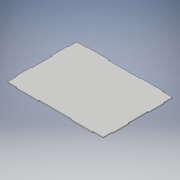
# Autodesk Inventor part: case_roof
Saved by Autodesk Inventor 2019 (Build 230136000, 136)
## iProperties
Created: 2019-07-12
Part Number: case_roof
Material: Generic
Document SubType Name: Modeling
Designer: Lino P
Density: 1 g/cm^3
Appearance: Default
Author: Lino P
Autodesk Inventor part; units mm, degrees
ref_plane "YZ Plane" through (0, 0, 0) normal (1, 0, 0) x (0, 1, 0)
ref_plane "XZ Plane" through (0, 0, 0) normal (0, 1, 0) x (-1, 0, 0)
ref_plane "XY Plane" through (0, 0, 0) normal (0, 0, 1) x (1, 0, 0)
sketch "Sketch1" plane through (0, 0, 0) normal (0, 0, 1) x (1, 0, 0)
  line L0 (0, 0) -> (27, 0)
  line L1 (27, 0) -> (27, 30.2)
  line L2 (27, 30.2) -> (0, 30.2)
  line L3 (0, 30.2) -> (0, 0)
  circle A0 centre (13.5, 15.1) radius 10.85
  circle A1 centre (4.1, 4.2) radius 1.3
  circle A2 centre (22.9, 26) radius 1.3
  line L4 (21.6, 26) -> (24.2, 26) construction
  line L5 (22.9, 26) -> (22.9, 27.3) construction
  line L6 (4.1, 4.2) -> (2.8, 4.2) construction
  line L7 (4.1, 4.2) -> (4.1, 2.9) construction
  line L8 (45, 0) -> (72, 0)
  line L9 (72, 0) -> (72, 30.2)
  line L10 (72, 30.2) -> (45, 30.2)
  line L11 (45, 30.2) -> (45, 0)
  circle A3 centre (58.5, 15.1) radius 10.85
  circle A4 centre (49.1, 4.2) radius 1.3
  circle A5 centre (67.9, 26) radius 1.3
  line L12 (66.6, 26) -> (69.2, 26) construction
  line L13 (67.9, 26) -> (67.9, 27.3) construction
  line L14 (49.1, 4.2) -> (47.8, 4.2) construction
  line L15 (49.1, 4.2) -> (49.1, 2.9) construction
  line L16 (90, 0) -> (117, 0)
  line L17 (117, 0) -> (117, 30.2)
  line L18 (117, 30.2) -> (90, 30.2)
  line L19 (90, 30.2) -> (90, 0)
  circle A6 centre (103.5, 15.1) radius 10.85
  circle A7 centre (94.1, 4.2) radius 1.3
  circle A8 centre (112.9, 26) radius 1.3
  line L20 (111.6, 26) -> (114.2, 26) construction
  line L21 (112.9, 26) -> (112.9, 27.3) construction
  line L22 (94.1, 4.2) -> (92.8, 4.2) construction
  line L23 (94.1, 4.2) -> (94.1, 2.9) construction
  line L24 (135, 0) -> (162, 0)
  line L25 (162, 0) -> (162, 30.2)
  line L26 (162, 30.2) -> (135, 30.2)
  line L27 (135, 30.2) -> (135, 0)
  circle A9 centre (148.5, 15.1) radius 10.85
  circle A10 centre (139.1, 4.2) radius 1.3
  circle A11 centre (157.9, 26) radius 1.3
  line L28 (156.6, 26) -> (159.2, 26) construction
  line L29 (157.9, 26) -> (157.9, 27.3) construction
  line L30 (139.1, 4.2) -> (137.8, 4.2) construction
  line L31 (139.1, 4.2) -> (139.1, 2.9) construction
  line L32 (180, 0) -> (207, 0)
  line L33 (207, 0) -> (207, 30.2)
  line L34 (207, 30.2) -> (180, 30.2)
  line L35 (180, 30.2) -> (180, 0)
  circle A12 centre (193.5, 15.1) radius 10.85
  circle A13 centre (184.1, 4.2) radius 1.3
  circle A14 centre (202.9, 26) radius 1.3
  line L36 (201.6, 26) -> (204.2, 26) construction
  line L37 (202.9, 26) -> (202.9, 27.3) construction
  line L38 (184.1, 4.2) -> (182.8, 4.2) construction
  line L39 (184.1, 4.2) -> (184.1, 2.9) construction
  line L40 (225, 0) -> (252, 0)
  line L41 (252, 0) -> (252, 30.2)
  line L42 (252, 30.2) -> (225, 30.2)
  line L43 (225, 30.2) -> (225, 0)
  circle A15 centre (238.5, 15.1) radius 10.85
  circle A16 centre (229.1, 4.2) radius 1.3
  circle A17 centre (247.9, 26) radius 1.3
  line L44 (246.6, 26) -> (249.2, 26) construction
  line L45 (247.9, 26) -> (247.9, 27.3) construction
  line L46 (229.1, 4.2) -> (227.8, 4.2) construction
  line L47 (229.1, 4.2) -> (229.1, 2.9) construction
  line L48 (270, 0) -> (297, 0)
  line L49 (297, 0) -> (297, 30.2)
  line L50 (297, 30.2) -> (270, 30.2)
  line L51 (270, 30.2) -> (270, 0)
  circle A18 centre (283.5, 15.1) radius 10.85
  circle A19 centre (274.1, 4.2) radius 1.3
  circle A20 centre (292.9, 26) radius 1.3
  line L52 (291.6, 26) -> (294.2, 26) construction
  line L53 (292.9, 26) -> (292.9, 27.3) construction
  line L54 (274.1, 4.2) -> (272.8, 4.2) construction
  line L55 (274.1, 4.2) -> (274.1, 2.9) construction
  line L56 (315, 0) -> (342, 0)
  line L57 (342, 0) -> (342, 30.2)
  line L58 (342, 30.2) -> (315, 30.2)
  line L59 (315, 30.2) -> (315, 0)
  circle A21 centre (328.5, 15.1) radius 10.85
  circle A22 centre (319.1, 4.2) radius 1.3
  circle A23 centre (337.9, 26) radius 1.3
  line L60 (336.6, 26) -> (339.2, 26) construction
  line L61 (337.9, 26) -> (337.9, 27.3) construction
  line L62 (319.1, 4.2) -> (317.8, 4.2) construction
  line L63 (319.1, 4.2) -> (319.1, 2.9) construction
  line L64 (0, -60) -> (27, -60)
  line L65 (27, -60) -> (27, -29.8)
  line L66 (27, -29.8) -> (0, -29.8)
  line L67 (0, -29.8) -> (0, -60)
  circle A24 centre (13.5, -44.9) radius 10.85
  circle A25 centre (4.1, -55.8) radius 1.3
  circle A26 centre (22.9, -34) radius 1.3
  line L68 (21.6, -34) -> (24.2, -34) construction
  line L69 (22.9, -34) -> (22.9, -32.7) construction
  line L70 (4.1, -55.8) -> (2.8, -55.8) construction
  line L71 (4.1, -55.8) -> (4.1, -57.1) construction
  line L72 (45, -60) -> (72, -60)
  line L73 (72, -60) -> (72, -29.8)
  line L74 (72, -29.8) -> (45, -29.8)
  line L75 (45, -29.8) -> (45, -60)
  circle A27 centre (58.5, -44.9) radius 10.85
  circle A28 centre (49.1, -55.8) radius 1.3
  circle A29 centre (67.9, -34) radius 1.3
  line L76 (66.6, -34) -> (69.2, -34) construction
  line L77 (67.9, -34) -> (67.9, -32.7) construction
  line L78 (49.1, -55.8) -> (47.8, -55.8) construction
  line L79 (49.1, -55.8) -> (49.1, -57.1) construction
  line L80 (90, -60) -> (117, -60)
  line L81 (117, -60) -> (117, -29.8)
  line L82 (117, -29.8) -> (90, -29.8)
  line L83 (90, -29.8) -> (90, -60)
  circle A30 centre (103.5, -44.9) radius 10.85
  circle A31 centre (94.1, -55.8) radius 1.3
  circle A32 centre (112.9, -34) radius 1.3
  line L84 (111.6, -34) -> (114.2, -34) construction
  line L85 (112.9, -34) -> (112.9, -32.7) construction
  line L86 (94.1, -55.8) -> (92.8, -55.8) construction
  line L87 (94.1, -55.8) -> (94.1, -57.1) construction
  line L88 (135, -60) -> (162, -60)
  line L89 (162, -60) -> (162, -29.8)
  line L90 (162, -29.8) -> (135, -29.8)
  line L91 (135, -29.8) -> (135, -60)
  circle A33 centre (148.5, -44.9) radius 10.85
  circle A34 centre (139.1, -55.8) radius 1.3
  circle A35 centre (157.9, -34) radius 1.3
  line L92 (156.6, -34) -> (159.2, -34) construction
  line L93 (157.9, -34) -> (157.9, -32.7) construction
  line L94 (139.1, -55.8) -> (137.8, -55.8) construction
  line L95 (139.1, -55.8) -> (139.1, -57.1) construction
  line L96 (180, -60) -> (207, -60)
  line L97 (207, -60) -> (207, -29.8)
  line L98 (207, -29.8) -> (180, -29.8)
  line L99 (180, -29.8) -> (180, -60)
  circle A36 centre (193.5, -44.9) radius 10.85
  circle A37 centre (184.1, -55.8) radius 1.3
  circle A38 centre (202.9, -34) radius 1.3
  line L100 (201.6, -34) -> (204.2, -34) construction
  line L101 (202.9, -34) -> (202.9, -32.7) construction
  line L102 (184.1, -55.8) -> (182.8, -55.8) construction
  line L103 (184.1, -55.8) -> (184.1, -57.1) construction
  line L104 (225, -60) -> (252, -60)
  line L105 (252, -60) -> (252, -29.8)
  line L106 (252, -29.8) -> (225, -29.8)
  line L107 (225, -29.8) -> (225, -60)
  circle A39 centre (238.5, -44.9) radius 10.85
  circle A40 centre (229.1, -55.8) radius 1.3
  circle A41 centre (247.9, -34) radius 1.3
  line L108 (246.6, -34) -> (249.2, -34) construction
  line L109 (247.9, -34) -> (247.9, -32.7) construction
  line L110 (229.1, -55.8) -> (227.8, -55.8) construction
  line L111 (229.1, -55.8) -> (229.1, -57.1) construction
  line L112 (270, -60) -> (297, -60)
  line L113 (297, -60) -> (297, -29.8)
  line L114 (297, -29.8) -> (270, -29.8)
  line L115 (270, -29.8) -> (270, -60)
  circle A42 centre (283.5, -44.9) radius 10.85
  circle A43 centre (274.1, -55.8) radius 1.3
  circle A44 centre (292.9, -34) radius 1.3
  line L116 (291.6, -34) -> (294.2, -34) construction
  line L117 (292.9, -34) -> (292.9, -32.7) construction
  line L118 (274.1, -55.8) -> (272.8, -55.8) construction
  line L119 (274.1, -55.8) -> (274.1, -57.1) construction
  line L120 (315, -60) -> (342, -60)
  line L121 (342, -60) -> (342, -29.8)
  line L122 (342, -29.8) -> (315, -29.8)
  line L123 (315, -29.8) -> (315, -60)
  circle A45 centre (328.5, -44.9) radius 10.85
  circle A46 centre (319.1, -55.8) radius 1.3
  circle A47 centre (337.9, -34) radius 1.3
  line L124 (336.6, -34) -> (339.2, -34) construction
  line L125 (337.9, -34) -> (337.9, -32.7) construction
  line L126 (319.1, -55.8) -> (317.8, -55.8) construction
  line L127 (319.1, -55.8) -> (319.1, -57.1) construction
  line L128 (-15, 60.2) -> (357, 60.2)
  line L129 (357, 60.2) -> (357, -80)
  line L130 (357, -80) -> (-15, -80)
  line L131 (-15, -80) -> (-15, 60.2)
  line L132 (7, 35.2) -> (20, 35.2)
  line L133 (20, 35.2) -> (20, 44.2)
  line L134 (20, 44.2) -> (7, 44.2)
  line L135 (7, 44.2) -> (7, 35.2)
  line L136 (7, 35.2) -> (20, 44.2) construction
  line L137 (20, 35.2) -> (7, 44.2) construction
  line L138 (65, 35.2) -> (65, 44.2)
  line L139 (52, 35.2) -> (65, 35.2)
  line L140 (65, 44.2) -> (52, 44.2)
  line L141 (65, 35.2) -> (52, 44.2) construction
  line L142 (52, 44.2) -> (52, 35.2)
  line L143 (52, 35.2) -> (65, 44.2) construction
  line L144 (110, 35.2) -> (110, 44.2)
  line L145 (97, 35.2) -> (110, 35.2)
  line L146 (110, 44.2) -> (97, 44.2)
  line L147 (110, 35.2) -> (97, 44.2) construction
  line L148 (97, 44.2) -> (97, 35.2)
  line L149 (97, 35.2) -> (110, 44.2) construction
  line L150 (155, 35.2) -> (155, 44.2)
  line L151 (142, 35.2) -> (155, 35.2)
  line L152 (155, 44.2) -> (142, 44.2)
  line L153 (155, 35.2) -> (142, 44.2) construction
  line L154 (142, 44.2) -> (142, 35.2)
  line L155 (142, 35.2) -> (155, 44.2) construction
  line L156 (200, 35.2) -> (200, 44.2)
  line L157 (187, 35.2) -> (200, 35.2)
  line L158 (200, 44.2) -> (187, 44.2)
  line L159 (200, 35.2) -> (187, 44.2) construction
  line L160 (187, 44.2) -> (187, 35.2)
  line L161 (187, 35.2) -> (200, 44.2) construction
  line L162 (245, 35.2) -> (245, 44.2)
  line L163 (232, 35.2) -> (245, 35.2)
  line L164 (245, 44.2) -> (232, 44.2)
  line L165 (245, 35.2) -> (232, 44.2) construction
  line L166 (232, 44.2) -> (232, 35.2)
  line L167 (232, 35.2) -> (245, 44.2) construction
  line L168 (290, 35.2) -> (290, 44.2)
  line L169 (277, 35.2) -> (290, 35.2)
  line L170 (290, 44.2) -> (277, 44.2)
  line L171 (290, 35.2) -> (277, 44.2) construction
  line L172 (277, 44.2) -> (277, 35.2)
  line L173 (277, 35.2) -> (290, 44.2) construction
  line L174 (335, 35.2) -> (335, 44.2)
  line L175 (322, 35.2) -> (335, 35.2)
  line L176 (335, 44.2) -> (322, 44.2)
  line L177 (335, 35.2) -> (322, 44.2) construction
  line L178 (322, 44.2) -> (322, 35.2)
  line L179 (322, 35.2) -> (335, 44.2) construction
  line L180 (20, -24.8) -> (20, -15.8)
  line L181 (7, -24.8) -> (20, -24.8)
  line L182 (20, -15.8) -> (7, -15.8)
  line L183 (20, -24.8) -> (7, -15.8) construction
  line L184 (7, -15.8) -> (7, -24.8)
  line L185 (7, -24.8) -> (20, -15.8) construction
  line L186 (65, -24.8) -> (65, -15.8)
  line L187 (52, -24.8) -> (65, -24.8)
  line L188 (65, -15.8) -> (52, -15.8)
  line L189 (65, -24.8) -> (52, -15.8) construction
  line L190 (52, -15.8) -> (52, -24.8)
  line L191 (52, -24.8) -> (65, -15.8) construction
  line L192 (110, -24.8) -> (110, -15.8)
  line L193 (97, -24.8) -> (110, -24.8)
  line L194 (110, -15.8) -> (97, -15.8)
  line L195 (110, -24.8) -> (97, -15.8) construction
  line L196 (97, -15.8) -> (97, -24.8)
  line L197 (97, -24.8) -> (110, -15.8) construction
  line L198 (155, -24.8) -> (155, -15.8)
  line L199 (142, -24.8) -> (155, -24.8)
  line L200 (155, -15.8) -> (142, -15.8)
  line L201 (155, -24.8) -> (142, -15.8) construction
  line L202 (142, -15.8) -> (142, -24.8)
  line L203 (142, -24.8) -> (155, -15.8) construction
  line L204 (200, -24.8) -> (200, -15.8)
  line L205 (187, -24.8) -> (200, -24.8)
  line L206 (200, -15.8) -> (187, -15.8)
  line L207 (200, -24.8) -> (187, -15.8) construction
  line L208 (187, -15.8) -> (187, -24.8)
  line L209 (187, -24.8) -> (200, -15.8) construction
  line L210 (245, -24.8) -> (245, -15.8)
  line L211 (232, -24.8) -> (245, -24.8)
  line L212 (245, -15.8) -> (232, -15.8)
  line L213 (245, -24.8) -> (232, -15.8) construction
  line L214 (232, -15.8) -> (232, -24.8)
  line L215 (232, -24.8) -> (245, -15.8) construction
  line L216 (290, -24.8) -> (290, -15.8)
  line L217 (277, -24.8) -> (290, -24.8)
  line L218 (290, -15.8) -> (277, -15.8)
  line L219 (290, -24.8) -> (277, -15.8) construction
  line L220 (277, -15.8) -> (277, -24.8)
  line L221 (277, -24.8) -> (290, -15.8) construction
  line L222 (335, -24.8) -> (335, -15.8)
  line L223 (322, -24.8) -> (335, -24.8)
  line L224 (335, -15.8) -> (322, -15.8)
  line L225 (335, -24.8) -> (322, -15.8) construction
  line L226 (322, -15.8) -> (322, -24.8)
  line L227 (322, -24.8) -> (335, -15.8) construction
  line L228 (-15, -9.9) -> (357, -9.9) construction
  line L229 (171, 60.2) -> (171, -80) construction
  line L230 (-15, 44.2) -> (-9, 44.2)
  line L231 (-9, 44.2) -> (-9, 4.2)
  line L232 (-9, 4.2) -> (-15, 4.2)
  line L233 (-15, 4.2) -> (-15, 44.2)
  line L234 (-15, -64) -> (-9, -64)
  line L235 (-9, -64) -> (-9, -24)
  line L236 (-9, -24) -> (-15, -24)
  line L237 (-15, -24) -> (-15, -64)
  line L238 (357, 44.2) -> (351, 44.2)
  line L239 (351, 44.2) -> (351, 4.2)
  line L240 (351, 4.2) -> (357, 4.2)
  line L241 (357, 4.2) -> (357, 44.2)
  line L242 (351, -64) -> (351, -24)
  line L243 (357, -64) -> (351, -64)
  line L244 (357, -24) -> (357, -64)
  line L245 (351, -24) -> (357, -24)
  line L246 (25, 60.2) -> (110, 60.2)
  line L247 (110, 60.2) -> (110, 57.2)
  line L248 (110, 57.2) -> (25, 57.2)
  line L249 (25, 57.2) -> (25, 60.2)
  line L250 (317, 60.2) -> (232, 60.2)
  line L251 (232, 60.2) -> (232, 57.2)
  line L252 (232, 57.2) -> (317, 57.2)
  line L253 (317, 57.2) -> (317, 60.2)
  line L254 (25, -80) -> (110, -80)
  line L255 (110, -80) -> (110, -77)
  line L256 (110, -77) -> (25, -77)
  line L257 (25, -77) -> (25, -80)
  line L258 (317, -77) -> (317, -80)
  line L259 (232, -80) -> (232, -77)
  line L260 (232, -77) -> (317, -77)
  line L261 (317, -80) -> (232, -80)
  point P0 (13.5, 39.7)
  point P1 (58.5, 39.7)
  point P2 (103.5, 39.7)
  point P3 (148.5, 39.7)
  point P4 (193.5, 39.7)
  point P5 (238.5, 39.7)
  point P6 (283.5, 39.7)
  point P7 (328.5, 39.7)
  point P8 (13.5, -20.3)
  point P9 (58.5, -20.3)
  point P10 (103.5, -20.3)
  point P11 (148.5, -20.3)
  point P12 (193.5, -20.3)
  point P13 (238.5, -20.3)
  point P14 (283.5, -20.3)
  point P15 (328.5, -20.3)
  dimension "d0" = 27
  dimension "d1" = 30.2
  dimension "d3" = 21.7
  dimension "d4" = 2.6
  dimension "d7" = 2.6
  dimension "d8" = 2.8
  dimension "d9" = 2.9
  dimension "d10" = 2.8
  dimension "d11" = 2.9
  dimension "d14" = 45
  dimension "d17" = 60
  dimension "d22" = 15
  dimension "d23" = 15
  dimension "d24" = 30
  dimension "d25" = 20
  dimension "d26" = 13
  dimension "d27" = 9
  dimension "d28" = 5
  dimension "d31" = 45
  dimension "d34" = 60
  dimension "d38" = 6
  dimension "d39" = 40
  dimension "d41" = 3
  dimension "d42" = 40
  dimension "d43" = 85
  constraints: 524 end point, 80 point on circle, 48 centre point, 35 midpoint, 24 symmetric about line, 10 parallel, 8 horizontal, 6 perpendicular, 3 vertical, 2 collinear, 2 point on line, 508 other
  measures "d0" distance of L2.end L1.end
  measures "d1" distance of L1.end L0.end
  measures "d3" diameter of A0
  measures "d4" diameter of A1
  measures "d7" diameter of A2
  measures "d8" distance from line of L1 L4.end
  measures "d9" distance from line of L2 L5.end
  measures "d10" distance from line of L3 L6.end
  measures "d11" distance from line of L0 L7.end
  measures "d14" distance of L1.end L9.end
  measures "d17" distance of L1.end L65.end
  measures "d22" distance between parallel lines of L131 L3
  measures "d23" distance between parallel lines of L57 L129
  measures "d24" distance between parallel lines of L18 L128
  measures "d25" distance between parallel lines of L72 L130
  measures "d26" distance of L134.end L133.end
  measures "d27" distance of L133.end L132.end
  measures "d28" distance between parallel lines of L2 L132
  measures "d31" distance of L132.end L138.start
  measures "d34" distance of L132.end L180.start
  measures "d38" distance of L231.end L232.end
  measures "d39" distance of L230.end L231.end
  measures "d41" distance of L246.end L247.end
  measures "d42" distance between parallel lines of L249 L131
  measures "d43" distance between parallel lines of L249 L247
ref_plane "Work Plane1" through (110, 60.2, 0) normal (0, 1, 0) x (1, 0, 0)
sketch "Sketch2" plane through (110, 60.2, 0) normal (0, 1, 0) x (1, 0, 0)
  line L0 (-85, -6) -> (-85, 0) projected
  line L1 (-85, 0) -> (-125, 0) construction
  line L2 (-125, 0) -> (-125, -6) construction
  line L3 (-85, -6) -> (-125, -6) construction
  line L4 (122, -6) -> (122, 0) projected
  line L5 (122, 0) -> (0, 0) construction
  line L6 (0, 0) -> (0, -6) projected
  line L7 (122, -6) -> (0, -6) construction
  line L8 (207, 0) -> (207, -6) projected
  line L9 (247, -6) -> (207, -6) construction
  line L10 (247, 0) -> (247, -6) construction
  line L11 (247, 0) -> (207, 0) construction
  line L12 (-85, 0) -> (-125, 0) projected
  line L13 (-122, 0) -> (244, 0)
  line L14 (244, 263.983) -> (-122, 263.983)
  line L15 (-125, 131.9915) -> (247, 131.9915) construction
  line L16 (61, 263.983) -> (61, 0) construction
  line L17 (-122, 263.983) -> (244, 263.983)
  line L18 (-85, -6) -> (-85, 269.983) construction
  line L19 (-85, 263.983) -> (0, 263.983)
  line L20 (0, 263.983) -> (0, 266.983)
  line L21 (0, 266.983) -> (-85, 266.983)
  line L22 (-85, 266.983) -> (-85, 263.983)
  line L23 (207, 263.983) -> (122, 263.983)
  line L24 (122, 263.983) -> (122, 266.983)
  line L25 (122, 266.983) -> (207, 266.983)
  line L26 (207, 266.983) -> (207, 263.983)
  line L27 (247, 34) -> (244, 34)
  line L28 (244, 34) -> (244, 94)
  line L29 (244, 94) -> (247, 94)
  line L30 (247, 94) -> (247, 34)
  line L31 (247, 229.983) -> (244, 229.983)
  line L32 (244, 229.983) -> (244, 169.983)
  line L33 (244, 169.983) -> (247, 169.983)
  line L34 (247, 169.983) -> (247, 229.983)
  line L35 (-125, 34) -> (-122, 34)
  line L36 (-122, 34) -> (-122, 94)
  line L37 (-122, 94) -> (-125, 94)
  line L38 (-125, 94) -> (-125, 34)
  line L39 (-125, 229.983) -> (-122, 229.983)
  line L40 (-122, 229.983) -> (-122, 169.983)
  line L41 (-122, 169.983) -> (-125, 169.983)
  line L42 (-125, 169.983) -> (-125, 229.983)
  line L43 (247, 34) -> (247, 94)
  line L44 (247, 169.983) -> (247, 229.983)
  line L45 (244, 169.983) -> (244, 94)
  line L46 (244, 229.983) -> (244, 263.983)
  line L47 (-125, 229.983) -> (-125, 169.983)
  line L48 (-125, 94) -> (-125, 34)
  line L49 (-122, 34) -> (-122, 0)
  line L50 (-122, 169.983) -> (-122, 94)
  line L51 (-122, 229.983) -> (-122, 263.983)
  line L52 (244, 34) -> (244, 0)
  line L53 (-85, 0) -> (0, 0)
  line L54 (0, 0) -> (0, -3)
  line L55 (0, -3) -> (-85, -3)
  line L56 (-85, -3) -> (-85, 0)
  line L57 (207, -3) -> (207, 0)
  line L58 (122, 0) -> (122, -3)
  line L59 (122, -3) -> (207, -3)
  line L60 (207, 0) -> (122, 0)
  point P0 (247, 263.983)
  point P1 (207, 269.983)
  dimension "d56" = 264
  dimension "d57" = 85
  dimension "d58" = 3
  dimension "d59" = 40
  dimension "d60" = 3
  dimension "d61" = 60
  constraints: 96 end point, 23 symmetric about line, 9 parallel, 7 perpendicular, 3 horizontal, 3 point on line, 3 vertical, 2 midpoint
  measures "d56" distance of L14.start point (247, 0)
  measures "d57" distance of L21.end L20.end
  measures "d58" distance of L20.end L19.end
  measures "d59" distance of L27.start L9.start
  measures "d60" distance of L29.end L28.end
  measures "d61" distance of L27.end L28.end
extrude "Extrusion6" add sketch "Sketch2" along normal blind 3
body "Solid2"
